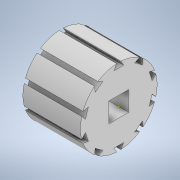
# Autodesk Inventor part: 220525 Large Rod Notched
Saved by Autodesk Inventor 2022 (Build 260153000, 153)
## iProperties
Created: 2022-05-25
Part Number: 220525 Large Rod Notched
Material: Generic
Document SubType Name: Modeling
Designer: josephinew
Density: 1 g/cm^3
Appearance: Default
Author: josephinew
Autodesk Inventor part; units mm, degrees
ref_plane "YZ Plane" through (0, 0, 0) normal (1, 0, 0) x (0, 1, 0)
ref_plane "XZ Plane" through (0, 0, 0) normal (0, 1, 0) x (-1, 0, 0)
ref_plane "XY Plane" through (0, 0, 0) normal (0, 0, 1) x (1, 0, 0)
sketch "Sketch1" plane through (0, 0, 0) normal (1, 0, 0) x (0, 1, 0)
  circle A0 centre (0, 0) radius 50.8
  line L0 (13.081, 13.081) -> (-13.081, 13.081)
  line L1 (-13.081, 13.081) -> (-13.081, -13.081)
  line L2 (-13.081, -13.081) -> (13.081, -13.081)
  line L3 (13.081, -13.081) -> (13.081, 13.081)
  point P0 (50.7268, 2.7261)
  point P1 (50.7268, -2.7261)
  dimension "d1" = 26.162
  dimension "d2" = 26.162
  constraints: 8 end point, 2 parallel, 2 point on circle, 1 centre point, 1 horizontal, 1 perpendicular
  measures "d1" distance of L2.end L1.end
  measures "d2" distance of L1.end L0.end
extrude "Extrusion2" add sketch "Sketch1" along normal blind 76.2
sketch "Sketch2" plane through (76.2, 0, 0) normal (1, 0, 0) x (0, 0, -1)
  line L0 (-6.35, 44.45) -> (-2.7261, 50.7268) projected
  line L1 (6.35, 44.45) -> (-6.35, 44.45) projected
  line L2 (-6.35, 44.45) -> (6.35, 44.45)
  line L3 (6.35, 44.45) -> (2.7261, 50.7268)
  line L4 (-6.35, 44.45) -> (-2.7261, 50.7268)
  arc A0 (2.7261, 50.7268) -> (-2.7261, 50.7268) centre (0, 0) ccw
  constraints: 6 end point, 2 point on circle, 1 centre point, 1 coincident, 1 horizontal
extrude "Extrusion3" cut sketch "Sketch2" against normal blind 76.2
pattern_circular "Circular Pattern1" count 10 over 360 about axis through (0, 0, 0) along (1, 0, 0) of "Extrusion3"
sketch "Sketch3" plane through (76.2, 0, 0) normal (1, 0, 0) x (0, 0, -1)
  point P0 (0, 0)
body "Solid2"
